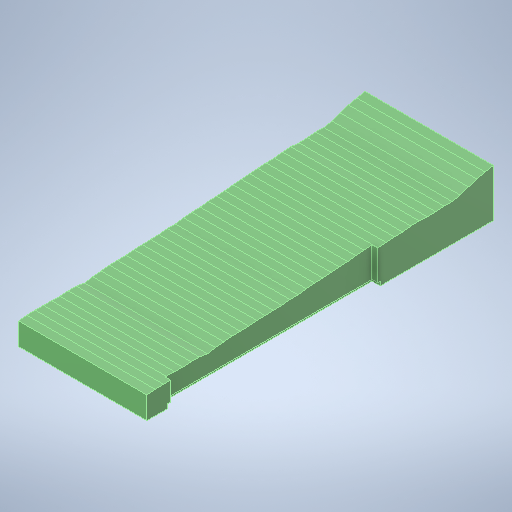
# Autodesk Inventor part: Elevation_Profile_Extending_NW_From_N_Edge_Of_Foundation_Where_Foundation_Meets_Ground
Saved by Autodesk Inventor 2025 (Build 290162010, 162A)
## iProperties
Created: 2024-08-02
Part Number: Elevation_Profile_Extending_NW_From_N_Edge_Of_Foundation_Where_Foundation_Meets_Ground
Material: Generic
Document SubType Name: Modeling
Designer: Tom
Density: 1 g/cm^3
Appearance: Smooth - Dark Forest Green
Author: Tom
Autodesk Inventor part; units mm, degrees
ref_plane "YZ Plane" through (0, 0, 0) normal (1, 0, 0) x (0, 1, 0)
ref_plane "XZ Plane" through (0, 0, 0) normal (0, 1, 0) x (-1, 0, 0)
sketch "Sketch1" plane through (0, 0, 0) normal (0, 1, 0) x (-1, 0, 0)
  line L0 (368.3, 1219.2) -> (368.3, -11582.4)
  line L1 (368.3, 1219.2) -> (336.55, 1219.2)
  line L2 (336.55, 1219.2) -> (279.4, 914.4)
  line L3 (279.4, 914.4) -> (209.55, 609.6)
  line L4 (209.55, 609.6) -> (107.95, 304.8)
  line L5 (107.95, 304.8) -> (0, 0)
  line L6 (0, 0) -> (-57.15, -299.3943)
  line L7 (-57.15, -299.3943) -> (-47.625, -604.0454)
  line L8 (-47.625, -604.0454) -> (-76.2, -907.503)
  line L9 (-76.2, -907.503) -> (-88.9, -1212.0383)
  line L10 (-88.9, -1212.0383) -> (-63.5, -1515.7781)
  line L11 (-63.5, -1515.7781) -> (-76.2, -1820.3134)
  line L12 (-76.2, -1820.3134) -> (-114.3, -2122.7228)
  line L13 (-114.3, -2122.7228) -> (-120.65, -2427.4566)
  line L14 (-120.65, -2427.4566) -> (-146.05, -2731.1964)
  line L15 (-146.05, -2731.1964) -> (-161.925, -3035.5828)
  line L16 (-161.925, -3035.5828) -> (-185.7375, -3339.4512)
  line L17 (-185.7375, -3339.4512) -> (-212.725, -3643.054)
  line L18 (-212.725, -3643.054) -> (-250.825, -3945.4634)
  line L19 (-250.825, -3945.4634) -> (-266.7, -4249.8497)
  line L20 (-266.7, -4249.8497) -> (-285.75, -4554.0538)
  line L21 (-285.75, -4554.0538) -> (-317.5, -4857.1957)
  line L22 (-317.5, -4857.1957) -> (-327.025, -5161.8468)
  line L23 (-327.025, -5161.8468) -> (-355.6, -5465.3044)
  line L24 (-355.6, -5465.3044) -> (-400.05, -5766.8458)
  line L25 (-400.05, -5766.8458) -> (-393.7, -6071.5797)
  line L26 (-393.7, -6071.5797) -> (-431.8, -6373.9891)
  line L27 (-431.8, -6373.9891) -> (-438.15, -6678.7229)
  line L28 (-438.15, -6678.7229) -> (-450.85, -6983.2582)
  line L29 (-450.85, -6983.2582) -> (-457.2, -7287.9921)
  line L30 (-457.2, -7287.9921) -> (-482.6, -7591.7319)
  line L31 (-482.6, -7591.7319) -> (-495.3, -7896.2672)
  line L32 (-495.3, -7896.2672) -> (-495.3, -8201.0672)
  line L33 (-495.3, -8201.0672) -> (-527.05, -8504.209)
  line L34 (-527.05, -8504.209) -> (-561.975, -8807.0015)
  line L35 (-561.975, -8807.0015) -> (-609.6, -9108.0578)
  line L36 (-609.6, -9108.0578) -> (-561.975, -9409.1141)
  line L37 (-561.975, -9409.1141) -> (-558.8, -9713.8976)
  line L38 (-558.8, -9713.8976) -> (-581.025, -10017.8862)
  line L39 (-581.025, -10017.8862) -> (-571.5, -10322.5373)
  line L40 (-571.5, -10322.5373) -> (-565.15, -10627.2712)
  line L41 (-565.15, -10627.2712) -> (-565.15, -10932.0712)
  line L42 (-565.15, -10932.0712) -> (-574.675, -11236.7223)
  line L43 (-574.675, -11236.7223) -> (-604.3377, -11540.0755)
  line L44 (-1422.4, 1219.2) -> (336.55, 1219.2)
  line L45 (-604.3377, -11540.0755) -> (-1422.4, -11540.0755)
  line L46 (-1422.4, -11540.0755) -> (-1422.4, 1219.2)
  point P0 (368.3, -5181.6)
  dimension "d4" = 1219.2
  dimension "d5" = 11582.4
  dimension "d6" = 368.3
  dimension "d8" = 31.75
  dimension "d10" = 304.8
  dimension "d14" = 88.9
  dimension "d15" = 304.8
  dimension "d16" = 304.8
  dimension "d17" = 260.35
  dimension "d18" = 158.75
  dimension "d20" = 304.8
  dimension "d21" = 425.45
  dimension "d22" = 304.8
  dimension "d23" = 415.925
  dimension "d24" = 304.8
  dimension "d25" = 444.5
  dimension "d26" = 304.8
  dimension "d27" = 457.2
  dimension "d28" = 304.8
  dimension "d29" = 431.8
  dimension "d30" = 304.8
  dimension "d31" = 444.5
  dimension "d32" = 304.8
  dimension "d33" = 482.6
  dimension "d34" = 304.8
  dimension "d35" = 488.95
  dimension "d36" = 304.8
  dimension "d37" = 514.35
  dimension "d39" = 304.8
  dimension "d40" = 530.225
  dimension "d41" = 304.8
  dimension "d42" = 554.0375
  dimension "d43" = 304.8
  dimension "d44" = 581.025
  dimension "d45" = 304.8
  dimension "d46" = 619.125
  dimension "d47" = 304.8
  dimension "d48" = 635
  dimension "d49" = 304.8
  dimension "d50" = 654.05
  dimension "d51" = 304.8
  dimension "d52" = 685.8
  dimension "d53" = 304.8
  dimension "d54" = 695.325
  dimension "d55" = 304.8
  dimension "d56" = 723.9
  dimension "d57" = 304.8
  dimension "d58" = 768.35
  dimension "d59" = 304.8
  dimension "d60" = 762
  dimension "d61" = 304.8
  dimension "d62" = 800.1
  dimension "d63" = 304.8
  dimension "d64" = 806.45
  dimension "d65" = 304.8
  dimension "d66" = 819.15
  dimension "d67" = 304.8
  dimension "d68" = 825.5
  dimension "d69" = 304.8
  dimension "d70" = 850.9
  dimension "d71" = 304.8
  dimension "d72" = 863.6
  dimension "d73" = 304.8
  dimension "d74" = 863.6
  constraints: 94 end point, 3 horizontal, 2 vertical, 1 midpoint
  measures "d4" vertical distance of L0.start L5.end
  measures "d5" vertical distance of L0.end L5.end
  measures "d6" distance from line of L0 L5.end
  measures "d8" distance of L0.start L1.end
  measures "d10" vertical distance of L1.end L2.end
  measures "d14" distance from line of L0 L2.end
  measures "d15" vertical distance of L3.end L2.end
  measures "d16" vertical distance of L4.end L3.end
  measures "d17" distance from line of L0 L4.end
  measures "d18" distance from line of L0 L3.end
  measures "d20" distance of L5.end L6.end
  measures "d21" distance from line of L0 L6.end
  measures "d22" distance of L6.end L7.end
  measures "d23" distance from line of L0 L7.end
  measures "d24" distance of L7.end L8.end
  measures "d25" distance from line of L0 L8.end
  measures "d26" distance of L8.end L9.end
  measures "d27" distance from line of L0 L9.end
  measures "d28" distance of L9.end L10.end
  measures "d29" distance from line of L0 L10.end
  measures "d30" distance of L10.end L11.end
  measures "d31" distance from line of L0 L11.end
  measures "d32" distance of L11.end L12.end
  measures "d33" distance from line of L0 L12.end
  measures "d34" distance of L12.end L13.end
  measures "d35" distance from line of L0 L13.end
  measures "d36" distance of L13.end L14.end
  measures "d37" distance from line of L0 L14.end
  measures "d39" distance of L14.end L15.end
  measures "d40" distance from line of L0 L15.end
  measures "d41" distance of L15.end L16.end
  measures "d42" distance from line of L0 L16.end
  measures "d43" distance of L16.end L17.end
  measures "d44" distance from line of L0 L17.end
  measures "d45" distance of L17.end L18.end
  measures "d46" distance from line of L0 L18.end
  measures "d47" distance of L18.end L19.end
  measures "d48" distance from line of L0 L19.end
  measures "d49" distance of L19.end L20.end
  measures "d50" distance from line of L0 L20.end
  measures "d51" distance of L20.end L21.end
  measures "d52" distance from line of L0 L21.end
  measures "d53" distance of L21.end L22.end
  measures "d54" horizontal distance of point (368.3, -5181.6) L22.end
  measures "d55" distance of L22.end L23.end
  measures "d56" distance from line of L0 L23.end
  measures "d57" distance of L23.end L24.end
  measures "d58" distance from line of L0 L24.end
  measures "d59" distance of L24.end L25.end
  measures "d60" distance from line of L0 L25.end
  measures "d61" distance of L25.end L26.end
  measures "d62" distance from line of L0 L26.end
  measures "d63" distance of L26.end L27.end
  measures "d64" distance from line of L0 L27.end
  measures "d65" distance of L27.end L28.end
  measures "d66" distance from line of L0 L28.end
  measures "d67" distance of L28.end L29.end
  measures "d68" distance from line of L0 L29.end
  measures "d69" distance of L29.end L30.end
  measures "d70" distance from line of L0 L30.end
  measures "d71" distance of L30.end L31.end
  measures "d72" distance from line of L0 L31.end
  measures "d73" distance of L31.end L32.end
  measures "d74" distance from line of L0 L32.end
extrude "Extrusion1" add sketch "Sketch1" along normal blind 4724.4
ref_plane "Work Plane1" through (0, 0, 0) normal (1, 0, 0) x (0, 1, 0)
sketch "Sketch2" plane through (0, 0, 0) normal (0, -1, 0) x (1, 0, 0)
  line L0 (1422.4, 1219.2) -> (1422.4, -11540.0755) projected
  line L1 (1422.4, -10769.6) -> (1270, -10769.6)
  line L2 (1270, -10769.6) -> (1270, -2946.4)
  line L3 (1270, -2946.4) -> (1422.4, -2946.4)
  line L4 (1422.4, -2946.4) -> (1422.4, -10769.6)
  point P0 (0, 0)
  dimension "d101" = 2946.4
  dimension "d102" = 152.4
  dimension "d103" = 7823.2
  constraints: 8 end point, 2 parallel, 1 horizontal, 1 perpendicular, 1 point on line
  measures "d101" distance from line of L3 point (0, 0)
  measures "d102" distance of L1.start L1.end
  measures "d103" distance of L1.end L2.end
extrude "Extrusion2" cut sketch "Sketch2" against normal blind 304.8
sketch "Sketch3" plane through (0, 0, 0) normal (0, -1, 0) x (1, 0, 0)
  line L0 (1270, -10668) -> (-142.875, -10668)
  line L1 (-142.875, -10668) -> (-142.875, -3048)
  line L2 (-142.875, -3048) -> (1270, -3048)
  line L3 (1270, -3048) -> (1270, -10668)
  line L4 (1422.4, -10769.6) -> (1270, -10769.6) projected
  line L5 (1270, -10769.6) -> (1270, -2946.4) projected
  line L6 (1270, -2946.4) -> (1422.4, -2946.4) projected
  line L7 (185.7375, -3339.4512) -> (161.925, -3035.5828) projected
  point P0 (0, 0)
  point P1 (162.8981, -3048)
  dimension "d106" = 101.6
  dimension "d107" = 101.6
  dimension "d111" = 1412.875
  constraints: 8 end point, 2 parallel, 2 point on line, 1 collinear, 1 horizontal, 1 perpendicular
  measures "d106" distance between parallel lines of L4 L0
  measures "d107" distance between parallel lines of L6 L2
  measures "d111" distance between parallel lines of L1 L3
extrude "Extrusion3" cut sketch "Sketch3" against normal blind 203.2
body "Solid1"
